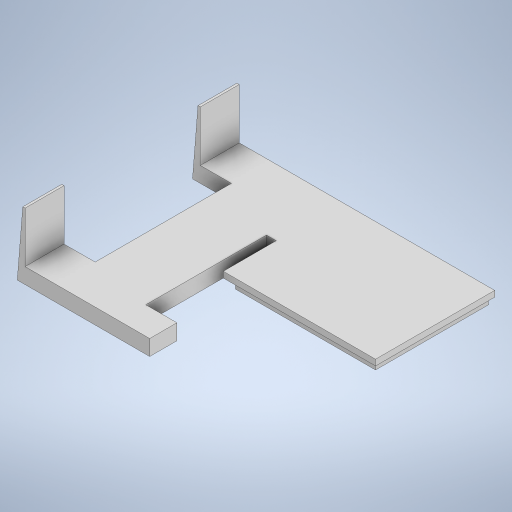
# Autodesk Inventor part: box_hut03_10_2025
Saved by Autodesk Inventor 2024.2 (Build 282272000, 272)
## iProperties
Created: 2025-09-01
Part Number: box_hut03_10_2025
Material: Типовые
Document SubType Name: Modeling
Designer: winds
Density: 1 g/cm^3
Appearance: По умолчанию
Author: winds
Autodesk Inventor part; units mm, degrees
ref_plane "YZ Plane" through (0, 0, 0) normal (1, 0, 0) x (0, 1, 0)
ref_plane "XZ Plane" through (0, 0, 0) normal (0, 1, 0) x (-1, 0, 0)
ref_plane "XY Plane" through (0, 0, 0) normal (0, 0, 1) x (1, 0, 0)
sketch "плоскость" plane through (0, 0, 0) normal (0, 1, 0) x (-1, 0, 0)
  line L0 (68, 55) -> (0, 55)
  line L1 (0, 55) -> (0, 0)
  line L2 (0, 0) -> (68, 0)
  line L3 (68, 0) -> (68, 55)
  dimension "d0" = 68
  dimension "d1" = 55
  constraints: 8 end point, 2 parallel, 1 horizontal, 1 perpendicular
  measures "d0" distance of L0.start L0.end
  measures "d1" distance of L0.end L1.end
extrude "толщина" add sketch "плоскость" along normal blind 4
sketch "вырез" plane through (0, 4, 0) normal (0, 1, 0) x (1, 0, 0)
  line L0 (-68, 0) -> (-68, -55) projected
  line L1 (-68, -45) -> (-58, -45)
  line L2 (-58, -45) -> (-58, -10)
  line L3 (-58, -10) -> (-68, -10)
  line L4 (-68, -10) -> (-68, -45)
  line L5 (0, -55) -> (0, 0) projected
  line L6 (-68, -55) -> (0, -55) projected
  line L7 (0, -31) -> (-42, -31)
  line L8 (-42, -31) -> (-42, -55)
  line L9 (-42, -55) -> (0, -55)
  line L10 (0, -55) -> (0, -31)
  line L11 (0, 0) -> (-68, 0) projected
  point P0 (-68, -10)
  point P1 (-63, -10)
  point P2 (-63, -45)
  dimension "d4" = 35
  dimension "d5" = 10
  dimension "d25" = 58
  dimension "d34" = 10
  dimension "d35" = 10
  constraints: 16 end point, 4 parallel, 3 point on line, 2 horizontal, 2 midpoint, 2 perpendicular
  measures "d4" distance of L1.end L2.end
  measures "d5" distance of L2.end L3.end
  measures "d25" distance between parallel lines of L5 L2
  measures "d34" distance from line of L11 point (-63, -10)
  measures "d35" distance from line of L6 point (-63, -45)
extrude "вырез глубина" cut sketch "вырез" against normal blind 4 contours L3 L2 L1 L0
sketch "Эскиз3" plane through (0, 4, 0) normal (0, 1, 0) x (1, 0, 0)
  line L0 (-68, 0) -> (-68, -55) projected
  line L1 (-58, -45) -> (-68, -45) projected
  line L2 (-68, -55) -> (-66, -55)
  line L3 (-66, -55) -> (-66, -45)
  line L4 (-66, -45) -> (-68, -45)
  line L5 (-68, -45) -> (-68, -55)
  line L6 (-58, -10) -> (-68, -10) projected
  line L7 (0, 0) -> (-68, 0) projected
  line L8 (-68, -10) -> (-66, -10)
  line L9 (-66, -10) -> (-66, 0)
  line L10 (-66, 0) -> (-68, 0)
  line L11 (-68, 0) -> (-68, -10)
  point P0 (-68, 0)
  constraints: 16 end point, 4 parallel, 2 horizontal, 2 perpendicular, 2 point on line
extrude "Выдавливание3" add sketch "Эскиз3" along normal blind 13
sketch "лапки" plane through (-68, 0, 55) normal (0, 0, 1) x (1, 0, 0)
  line L0 (0, 0) -> (0, 17) projected
  line L1 (0, 0) -> (0, 17)
  line L2 (0, 17) -> (1.41, 17)
  line L3 (0, 0) -> (10, 0) projected
  line L4 (1.41, 17) -> (0, 0)
  point P0 (68, 0)
  point P1 (0, 1)
  point P2 (0, 1)
  constraints: 6 end point, 1 collinear, 1 perpendicular
extrude "Выдавливание4" cut sketch "лапки" against normal through all
sketch "Эскиз10" plane through (0, 4, 0) normal (0, 1, 0) x (1, 0, 0)
  line L0 (0, -55) -> (0, 0) projected
  line L1 (-68, -55) -> (0, -55) projected
  line L2 (0, -31) -> (-42, -31)
  line L3 (-42, -31) -> (-42, -55)
  line L4 (-42, -55) -> (0, -55)
  line L5 (0, -55) -> (0, -31)
  constraints: 8 end point, 2 parallel, 2 point on line, 1 horizontal, 1 perpendicular
extrude "Выдавливание7" cut sketch "Эскиз10" against normal blind 4
sketch "Эскиз11" plane through (0, 4, 0) normal (0, 1, 0) x (1, 0, 0)
  line L0 (0, -31) -> (-42, -31) projected
  line L1 (-40, -17) -> (-42, -17)
  line L2 (-42, -17) -> (-42, -31)
  line L3 (-42, -31) -> (-40, -31)
  line L4 (-40, -31) -> (-40, -17)
  point P0 (0, 0)
  constraints: 8 end point, 2 parallel, 1 horizontal, 1 perpendicular
extrude "Выдавливание8" cut sketch "Эскиз11" against normal blind 4
sketch "Эскиз12" plane through (0, 4, 0) normal (0, 1, 0) x (1, 0, 0)
  line L0 (-42, -55) -> (-42, -17) projected
  line L1 (-42, -48) -> (-34, -48)
  line L2 (-34, -48) -> (-34, -55)
  line L3 (-34, -55) -> (-42, -55)
  line L4 (-42, -55) -> (-42, -48)
  line L5 (-40, -31) -> (0, -31) projected
  point P0 (0, 0)
  point P1 (-42, -55)
  point P2 (-38, -55)
  point P3 (-38, -48)
  point P4 (-42, -51.5)
  point P5 (-34, -51.5)
  dimension "d36" = 7
  dimension "d37" = 8
  dimension "d38" = 17
  constraints: 8 end point, 4 midpoint, 2 parallel, 1 horizontal, 1 perpendicular, 1 point on line
  measures "d36" distance of point (-38, -55) point (-38, -48)
  measures "d37" distance of point (-42, -51.5) point (-34, -51.5)
  measures "d38" distance between parallel lines of L1 L5
extrude "Выдавливание9" add sketch "Эскиз12" against normal blind 4
sketch "Эскиз14" plane through (0, 0, 0) normal (0, -1, 0) x (1, 0, 0)
  line L0 (-42, 17) -> (-40, 17) projected
  line L1 (-40, 17) -> (-38, 17)
  line L2 (-38, 17) -> (-38, 31)
  line L3 (-38, 31) -> (-40, 31)
  line L4 (-40, 31) -> (-40, 17)
  line L5 (0, 31) -> (0, 0) projected
  line L6 (-40, 29) -> (0, 29)
  line L7 (0, 29) -> (0, 31)
  line L8 (0, 31) -> (-40, 31)
  line L9 (-40, 31) -> (-40, 29)
  line L10 (0, 0) -> (-68, 0) projected
  line L11 (0, 31) -> (-2, 31)
  line L12 (-2, 31) -> (-2, 0)
  line L13 (-2, 0) -> (0, 0)
  line L14 (0, 0) -> (0, 31)
  point P0 (-38, 29)
  point P1 (-2, 29)
  point P2 (-40, 24)
  point P3 (-38, 24)
  dimension "d46" = 2
  dimension "d47" = 2
  dimension "d48" = 2
  constraints: 24 end point, 6 parallel, 3 horizontal, 3 perpendicular, 2 midpoint, 2 point on line
  measures "d46" distance between parallel lines of L12 L5
  measures "d47" distance between parallel lines of L8 L6
  measures "d48" distance of point (-40, 24) point (-38, 24)
extrude "Выдавливание10" cut sketch "Эскиз14" against normal blind 2.5
sketch "Эскиз15" plane through (0, 2.5, 0) normal (0, -1, 0) x (1, 0, 0)
  line L0 (-40, 31) -> (0, 31) projected
  line L1 (0, 0) -> (-0.4, 0)
  line L2 (-0.4, 0) -> (-0.4, 31)
  line L3 (-0.4, 31) -> (0, 31)
  line L4 (0, 31) -> (0, 0)
  line L5 (-40, 17) -> (-40, 31) projected
  line L6 (0, 31) -> (-40, 31)
  line L7 (-40, 31) -> (-40, 30.6)
  line L8 (-40, 30.6) -> (0, 30.6)
  line L9 (0, 30.6) -> (0, 31)
  line L10 (-38, 17) -> (-42, 17) projected
  line L11 (-40, 31) -> (-39.5, 31)
  line L12 (-39.5, 31) -> (-39.5, 17)
  line L13 (-39.5, 17) -> (-40, 17)
  line L14 (-40, 17) -> (-40, 31)
  point P0 (0, 31)
  point P1 (-39.5, 30.6)
  point P2 (-0.4, 30.6)
  dimension "d41" = 0.4
  dimension "d42" = 0.4
  dimension "d43" = 0.5
  constraints: 24 end point, 6 parallel, 3 horizontal, 3 perpendicular, 3 point on line
  measures "d41" distance between parallel lines of L2 L4
  measures "d42" distance between parallel lines of L0 L8
  measures "d43" distance between parallel lines of L5 L12
extrude "Выдавливание11" cut sketch "Эскиз15" against normal blind 1.5
